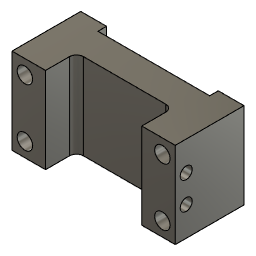
3020Table_ChipShouterAdapter_HardwareNeeded (Autodesk Fusion 360 design; units mm, degrees)
Autodesk Fusion 360 part; units mm, degrees
sketch "Sketch1" plane through (0, 0, 0) normal (0, 1, 0) x (1, 0, 0)
  line L0 (0, 0) -> (65, 0)
  line L1 (65, 0) -> (65, 5)
  line L2 (65, 5) -> (80, 5)
  line L3 (80, 5) -> (80, -35)
  line L4 (80, -35) -> (0, -35)
  line L5 (0, -35) -> (-15, -35)
  line L6 (-15, -35) -> (-15, 5)
  line L7 (-15, 5) -> (0, 5)
  line L8 (0, 5) -> (0, 0)
  line L9 (32.5, 0) -> (32.5, -35) construction
  line L10 (32.5, 0) -> (4.5, 0) construction
  line L11 (32.5, 0) -> (60.5, 0) construction
  line L12 (60.5, 0) -> (60.5, -17) construction
  line L13 (56.5, -17) -> (8.5, -17)
  line L14 (4.5, -21) -> (4.5, -35)
  line L15 (60.5, -21) -> (60.5, -35)
  arc A0 (8.5, -17) -> (4.5, -21) centre (8.5, -21) ccw
  arc A1 (60.5, -21) -> (56.5, -17) centre (56.5, -21) ccw
  point P0 (4.5, -17)
  dimension "d1" = 65
  dimension "d2" = 28
  dimension "d3" = 28
  dimension "d4" = 17
  dimension "d5" = 56
  dimension "d6" = 4
  dimension "d7" = 4
  constraint coincident L0.start L8.end
  constraint horizontal L0
  constraint perpendicular L0 L1
  constraint perpendicular L1 L2
  constraint perpendicular L2 L3
  constraint perpendicular L3 L4
  constraint perpendicular L3 L5
  constraint perpendicular L5 L6
  constraint perpendicular L6 L7
  constraint perpendicular L0 L8
  constraint midpoint L0 L9.start
  constraint coincident L4 L9.end
  constraint perpendicular L4 L9
  constraint perpendicular L9 L10
  constraint perpendicular L9 L11
  constraint perpendicular L11 L12
  constraint perpendicular L9 L13
  constraint coincident L4 L14.end
  constraint perpendicular L4 L14
  constraint coincident L4 L15.end
  constraint perpendicular L13 L15
  constraint coincident P0 L14
  constraint coincident P0 L13
  constraint tangent L14 A0
  constraint tangent L13 A0
  constraint coincident L12.end L13
  constraint coincident L12.end L15
  constraint tangent L13 A1
  constraint tangent L15 A1
  measures "d1" distance of L0.start L0.end
  measures "d2" distance of L9.start L10.end
  measures "d3" distance of L9.start L11.end
  measures "d4" distance of L11.end L12.end
  measures "d5" distance of L12.end P0
  measures "d6" radius of A0
  measures "d7" radius of A1
extrude "Extrude1" add sketch "Sketch1" along normal blind 50 contours L0 L1 L2 L3 L4 L5 L6 L7 L8 L13 L14 L15 A0 A1
sketch "Sketch2" plane through (0, 0, 35) normal (0, 0, 1) x (1, 0, 0)
  line L0 (-15, 0) -> (4.5, 0)
  line L1 (4.5, 0) -> (4.5, 50)
  line L2 (4.5, 50) -> (-15, 50)
  line L3 (-15, 50) -> (-15, 0)
  line L4 (-15, 25) -> (80, 25) construction
  line L5 (32.5, 0.0866) -> (32.5, 50) construction
  line L6 (32.5, 25) -> (72.5, 25) construction
  line L7 (72.5, 25) -> (72.5, 41.75) construction
  line L8 (72.5, 25) -> (72.5, 8.25) construction
  line L9 (72.5, 41.75) -> (-7.5, 41.75) construction
  line L10 (72.5, 8.25) -> (-7.5, 8.25) construction
  point P0 (-7.5, 41.75)
  point P1 (72.5, 41.75)
  point P2 (72.5, 8.25)
  point P3 (-7.5, 8.25)
  dimension "d10" = 40
  dimension "d11" = 16.75
  dimension "d12" = 16.75
  dimension "d13" = 80
  dimension "d14" = 80
  constraint midpoint L3 L4.start
  constraint perpendicular L3 L4
  constraint perpendicular L4 L5
  constraint midpoint L4 L6.start
  constraint perpendicular L5 L6
  constraint perpendicular L4 L7
  constraint perpendicular L6 L8
  constraint perpendicular L7 L9
  constraint perpendicular L8 L10
  constraint coincident P0 L9.end
  constraint coincident P1 L7.end
  constraint coincident P2 L8.end
  constraint coincident P3 L10.end
  measures "d10" distance of L6.start L6.end
  measures "d11" distance of L6.end P1
  measures "d12" distance of L6.end P2
  measures "d13" distance of P1 P0
  measures "d14" distance of P2 P3
hole "Hole1" at (-7.5, 41.75, 35) at (72.5, 41.75, 35) at (72.5, 8.25, 35) at (-7.5, 8.25, 35) direction (0, 0, -1) diameter 5.5 depth 40 tip angle 118 counterbore diameter 9 counterbore depth 22
sketch "Sketch3" plane through (80, 0, 0) normal (1, 0, 0) x (0, 0, -1)
  line L0 (-35, 0) -> (5, 0)
  line L1 (5, 0) -> (5, 50)
  line L2 (5, 50) -> (-35, 50)
  line L3 (-35, 50) -> (-35, 0)
  line L4 (5, 25) -> (-35, 25) construction
  line L5 (-28.6189, 25) -> (-28.6189, 33) construction
  line L6 (-28.6189, 33) -> (-28.6189, 17) construction
  point P0 (-28.6189, 33)
  point P1 (-28.6189, 17)
  constraint midpoint L1 L4.start
  constraint midpoint L3 L4.end
  constraint coincident L4 L5.start
  constraint perpendicular L4 L5
  constraint perpendicular L4 L6
  constraint coincident P0 L5.end
  constraint coincident P1 L6.end
hole "Hole2" at (80, 17, 28.6189) at (80, 33, 28.6189) direction (-1, 0, 0) diameter 4.9 depth 40 tip angle 118 counterbore diameter 7 counterbore depth 10
